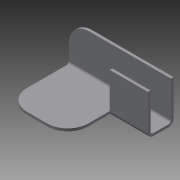
# Autodesk Inventor part: Igus Flange
Saved by Autodesk Inventor 2015 (Build 190159000, 159)
## iProperties
Created: 2015-02-08
Part Number: Igus Flange
Material: Generic
Document SubType Name: Sheet Metal
Designer: chapale16
Density: 1 g/cm^3
Flat Pattern Width: 12.7 cm
Flat Pattern Length: 12.6054 cm
Flat Pattern Area: 160.088 cm^2
Sheet Metal Rule: Default
Sheet Metal Width: 5.000 in
Sheet Metal Length: 4.963 in
Sheet Metal Area: 24.814 in^2
Appearance: Default
Author: chapale16
Autodesk Inventor part; units mm, degrees
ref_plane "YZ Plane" through (0, 0, 0) normal (1, 0, 0) x (0, 1, 0)
ref_plane "XZ Plane" through (0, 0, 0) normal (0, 1, 0) x (-1, 0, 0)
ref_plane "XY Plane" through (0, 0, 0) normal (0, 0, 1) x (1, 0, 0)
sketch "Sketch1" plane through (0, 0, 0) normal (0, 1, 0) x (-1, 0, 0)
  line L0 (0, 0) -> (127, 0)
  line L1 (127, 0) -> (127, 80.772)
  line L2 (127, 80.772) -> (0, 80.772)
  line L3 (0, 80.772) -> (0, 0)
  dimension "d0" = 127
  dimension "d1" = 80.772
  measures "d0" distance of L2.end L1.end
  measures "d1" distance of L1.end L0.end
extrude "Plate1" add sketch "Sketch1" along normal blind 3.175
sketch "Sketch2" plane through (-127, 0, 3.175) normal (0, 0, -1) x (-1, 0, 0)
  line L0 (-127, 0) -> (0, 0)
  line L1 (0, 0) -> (0, 50.8)
  line L2 (0, 50.8) -> (-127, 50.8)
  line L3 (-127, 50.8) -> (-127, 0)
  constraints: 6 end point, 1 horizontal, 1 perpendicular, 1 vertical
edge flange "Flange1" height 50.8 angle 90 thickness 3.175 bend radius 3.175 thickness toward (0, 0, -1) relief straight relief width 3.175 relief depth 1.5875 edges at (-63.5, 3.175, 0) wall of the first edge with corners at (0, 0, 3.175) (-127, 0, 3.175) (-127, 50.8, 3.175) (0, 50.8, 3.175)
bend "Bend1"
corner "Corner1"
sketch "Sketch4" plane through (0, 3.175, 0) normal (0, 1, 0) x (1, 0, 0)
  line L0 (0, -80.772) -> (0, -31.8516)
  line L1 (0, -6.35) -> (0, -80.772) projected
  line L2 (0, -31.8516) -> (-50.8, -31.8516)
  line L3 (-50.8, -31.8516) -> (-50.8, -80.772)
  line L4 (0, -80.772) -> (-127, -80.772) projected
  line L5 (0, -80.772) -> (-50.8, -80.772)
  point P0 (0, 0)
  dimension "d13" = 48.9204
  dimension "d14" = 50.8
  constraints: 8 end point, 3 perpendicular, 2 point on line
  measures "d13" distance of L0.start L0.end
  measures "d14" distance of L0.end L2.end
extrude "Cut1" cut sketch "Sketch4" against normal blind 3.175
sketch "Sketch5" plane through (0, 0, 28.6766) normal (0, 0, 1) x (1, 0, 0)
  line L0 (-47.625, 0) -> (0, 0)
  line L1 (0, 0) -> (0, 50.8)
  line L2 (0, 50.8) -> (-47.625, 50.8)
  line L3 (-47.625, 50.8) -> (-47.625, 0)
  constraints: 6 end point, 1 horizontal, 1 perpendicular, 1 vertical
edge flange "Flange2" height 50.8 angle 90 thickness 3.175 bend radius 3.175 thickness toward (0, 0, 1) relief straight relief width 3.175 relief depth 1.5875 edges at (-25.4, 3.175, 31.8516) wall of the first edge with corners at (-47.625, 0, 28.6766) (0, 0, 28.6766) (0, 50.8, 28.6766) (-47.625, 50.8, 28.6766)
bend "Bend2"
corner "Corner2"
fillet "Corner Round1" radius 25.4 2 edges at (-127, 1.5875, 80.772) (-50.8, 1.5875, 80.772)
fillet "Corner Round2" radius 25.4 1 edges at (-127, 50.8, 1.5875)
equation "\"d15\" = Thickness"
equation "\"d3\" = BendReliefWidth"
equation "\"d4\" = BendReliefDepth"
equation "\"d5\" = MinimumRemnant"
equation "\"d6\" = BendRadius"
equation "\"d9\" = BendRadius"
equation "\"d10\" = CornerReliefSize"
equation "\"d11\" = GapSize"
equation "\"d12\" = JacobiRadiusSize"
equation "\"d17\" = BendReliefWidth"
equation "\"d18\" = BendReliefDepth"
equation "\"d19\" = MinimumRemnant"
equation "\"d20\" = BendRadius"
equation "\"d23\" = BendRadius"
equation "\"d24\" = CornerReliefSize"
equation "\"d25\" = GapSize"
equation "\"d26\" = JacobiRadiusSize"
equation "\"BendRadius\" = Thickness"
equation "\"BendReliefWidth\" = Thickness"
equation "\"BendReliefDepth\" = 0.5 * Thickness"
equation "\"CornerReliefSize\" = 4 * Thickness"
equation "\"MinimumRemnant\" = 2 * Thickness"
equation "\"TransitionRadius\" = BendRadius"
equation "\"JacobiRadiusSize\" = BendRadius"
equation "\"GapSize\" = Thickness"
equation "\"d2\" = BendRadius"
equation "\"Thickness\" = 3.175"
body "Solid1"
